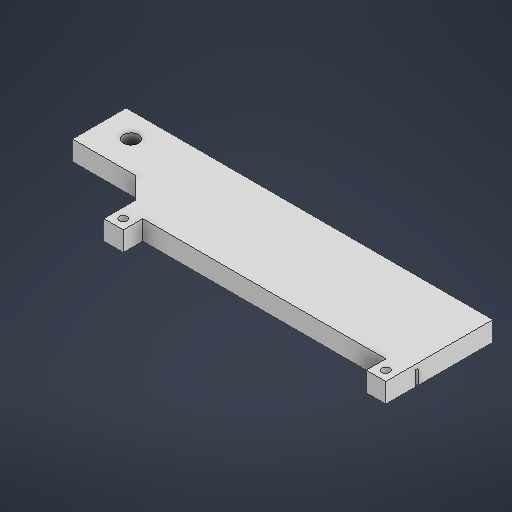
# Autodesk Inventor part: backwall
Saved by Autodesk Inventor 2025 (Build 290162000, 162)
## iProperties
Created: 2024-09-02
Part Number: backwall
Material: Generic
Document SubType Name: Modeling
Designer: Windows 7 was better
Density: 1 g/cm^3
Appearance: Default
Author: Windows 7 was better
Autodesk Inventor part; units mm, degrees
ref_plane "YZ Plane" through (0, 0, 0) normal (1, 0, 0) x (0, 1, 0)
ref_plane "XZ Plane" through (0, 0, 0) normal (0, 1, 0) x (-1, 0, 0)
ref_plane "XY Plane" through (0, 0, 0) normal (0, 0, 1) x (1, 0, 0)
sketch "Sketch1" plane through (0, 0, 0) normal (0, 1, 0) x (-1, 0, 0)
  line L0 (0, 0) -> (0, -20)
  line L1 (0, -20) -> (-150, -20)
  line L2 (-150, -20) -> (-150, 2)
  line L3 (-115.3934, 10.6066) -> (-34.6066, 10.6066)
  line L4 (-12, 0) -> (-12, -10) construction
  circle A0 centre (-12, -10) radius 3.1
  line L5 (-115.3934, 10.6066) -> (-150, 10.6066)
  line L6 (-150, 10.6066) -> (-150, 2)
  line L7 (0, 0) -> (0, 2)
  line L8 (-34.6066, 10.6066) -> (-26, 2)
  line L9 (-34.6066, 10.6066) -> (-22.435, 10.6066) construction
  line L10 (-26, 2) -> (0, 2)
  dimension "d3" = 20
  dimension "d4" = 150
  dimension "d7" = 10
  dimension "d8" = 6.2
  dimension "d17" = 2
  dimension "d18" = 45
  constraints: 22 end point, 3 horizontal, 2 parallel, 2 perpendicular, 2 vertical, 1 centre point, 1 coincident, 1 collinear, 1 equal length
  measures "d3" distance of L0.start L0.end
  measures "d4" distance of L0.end L1.end
  measures "d7" distance of L4.start L4.end
  measures "d8" diameter of A0
  measures "d17" distance of L0.start L7.end
  measures "d18" angle of L8 L9
extrude "Extrusion1" add sketch "Sketch1" along normal blind 6
sketch "Sketch2" plane through (0, 6, 0) normal (0, 1, 0) x (1, 0, 0)
  line L0 (24, 0) -> (34.6066, -10.6066) projected
  line L1 (34.6066, -10.6066) -> (150, -10.6066)
  line L2 (150, -10.6066) -> (150, -11.8066)
  line L3 (150, -11.8066) -> (34.6066, -11.8066)
  line L4 (34.6066, -11.8066) -> (34.6066, -10.6066)
  line L5 (34.6066, -10.6066) -> (150, -10.6066) projected
  line L6 (150, -10.6066) -> (150, 20) projected
  line L7 (150, 20) -> (0, 20) projected
  line L8 (0, 20) -> (0, -2) projected
  circle A0 centre (12, 10) radius 3.1 projected
  line L9 (0, -2) -> (26, -2) projected
  line L10 (26, -2) -> (34.6066, -10.6066) projected
  point P0 (0, 0)
  dimension "d11" = 1.2
  constraints: 8 end point, 2 parallel, 1 horizontal, 1 perpendicular
  measures "d11" distance of L1.end L2.end
extrude "Extrusion2" add sketch "Sketch2" along normal blind 2
sketch "Sketch3" plane through (0, 8, 0) normal (0, 1, 0) x (1, 0, 0)
  line L0 (34.6066, -11.8066) -> (150, -11.8066) projected
  line L1 (34.6066, -11.8066) -> (150, -11.8066)
  line L2 (150, -11.8066) -> (150, -15.8066)
  line L3 (150, -15.8066) -> (34.6066, -15.8066)
  line L4 (34.6066, -15.8066) -> (34.6066, -11.8066)
  point P0 (0, 0)
  dimension "d14" = 4
  constraints: 8 end point, 2 parallel, 1 horizontal, 1 perpendicular
  measures "d14" distance of L1.end L2.end
extrude "Extrusion3" add sketch "Sketch3" against normal up to surface (8 mm away)
sketch "Sketch4" plane through (0, 8, 0) normal (0, 1, 0) x (1, 0, 0)
  line L0 (34.6066, -15.8066) -> (150, -15.8066) projected
  line L1 (34.6066, -15.8066) -> (42.6066, -15.8066)
  line L2 (42.6066, -15.8066) -> (42.6066, -23.8066)
  line L3 (42.6066, -23.8066) -> (34.6066, -23.8066)
  line L4 (34.6066, -23.8066) -> (34.6066, -15.8066)
  line L5 (150, -15.8066) -> (142, -15.8066)
  line L6 (142, -15.8066) -> (142, -23.8066)
  line L7 (142, -23.8066) -> (150, -23.8066)
  line L8 (150, -23.8066) -> (150, -15.8066)
  circle A0 centre (38.6066, -19.8066) radius 1.6
  circle A1 centre (146, -19.8066) radius 1.6
  point P0 (0, 0)
  dimension "d19" = 8
  dimension "d20" = 8
  dimension "d21" = 8
  dimension "d22" = 8
  dimension "d23" = 3.2
  dimension "d24" = 3.2
  constraints: 16 end point, 4 parallel, 2 centre point, 2 horizontal, 2 perpendicular
  measures "d19" distance of L2.end L3.end
  measures "d20" distance of L1.end L2.end
  measures "d21" distance of L7.end L6.end
  measures "d22" distance of L6.end L5.end
  measures "d23" diameter of A0
  measures "d24" diameter of A1
extrude "Extrusion4" add sketch "Sketch4" against normal up to surface (8 mm away)
body "Solid1"
